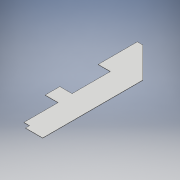
# Autodesk Inventor part: Gearbox-Side Cover Part 2
Saved by Autodesk Inventor 2018 (Build 220112000, 112)
## iProperties
Created: 2018-08-07
Part Number: Gearbox-Side Cover Part 2
Material: Generic
Document SubType Name: Modeling
Designer: P301319
Density: 1 g/cm^3
Appearance: Default
Author: P301319
Autodesk Inventor part; units mm, degrees
ref_plane "YZ Plane" through (0, 0, 0) normal (1, 0, 0) x (0, 1, 0)
ref_plane "XZ Plane" through (0, 0, 0) normal (0, 1, 0) x (-1, 0, 0)
ref_plane "XY Plane" through (0, 0, 0) normal (0, 0, 1) x (1, 0, 0)
sketch "Sketch1" plane through (0, 0, 0) normal (0, 0, 1) x (1, 0, 0)
  line L0 (0, 0) -> (0, 240)
  line L1 (0, 0) -> (75, 0)
  line L2 (0, 240) -> (34, 240)
  line L3 (34, 240) -> (220, 54)
  line L4 (34, 240) -> (338.7516, 240) construction
  line L5 (75, 0) -> (75, -235)
  line L6 (75, -235) -> (0, -235)
  line L7 (0, -235) -> (0, -325)
  line L8 (0, -325) -> (80, -325)
  line L9 (80, -325) -> (80, -535)
  line L10 (80, -535) -> (115, -535)
  line L11 (115, -535) -> (115, -560)
  line L12 (115, -560) -> (220, -560)
  line L13 (220, -560) -> (220, 54)
  dimension "d0" = 240
  dimension "d1" = 75
  dimension "d3" = 45
  dimension "d4" = 235
  dimension "d5" = 75
  dimension "d6" = 90
  dimension "d7" = 80
  dimension "d8" = 210
  dimension "d9" = 35
  dimension "d10" = 25
  dimension "d14" = 220
  dimension "d16" = 34
  constraints: 28 end point, 6 horizontal, 4 vertical, 3 perpendicular
  measures "d0" distance of L0.start L0.end
  measures "d1" distance of L0.start L1.end
  measures "d3" angle of L3 L4
  measures "d4" distance of L1.end L5.end
  measures "d5" distance of L5.end L6.end
  measures "d6" distance of L6.end L7.end
  measures "d7" distance of L7.end L8.end
  measures "d8" distance of L8.end L9.end
  measures "d9" distance of L9.end L10.end
  measures "d10" distance of L10.end L11.end
  measures "d14" distance between parallel lines of L0 L13
  measures "d16" distance of L0.end L2.end
extrude "Extrusion1" add sketch "Sketch1" along normal blind 1.6
equation "\"d5\" = d1"
body "Solid1"
